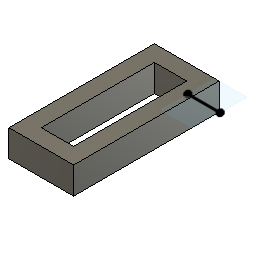
Teste+Medidor (Autodesk Fusion 360 design; units mm, degrees)
Autodesk Fusion 360 part; units mm, degrees
sketch "Esboço1" plane through (0, 0, 0) normal (0, 0, 1) x (1, 0, 0)
  line L0 (0, 0) -> (28.4, 0)
  line L1 (28.4, 0) -> (28.4, 58.2)
  line L2 (28.4, 58.2) -> (0, 58.2)
  line L3 (0, 58.2) -> (0, 0)
  line L4 (-5.0078, -5.0078) -> (33.4078, -5.0078)
  line L5 (33.4078, -5.0078) -> (33.4078, 63.2078)
  line L6 (33.4078, 63.2078) -> (-5.0078, 63.2078)
  line L7 (-5.0078, 63.2078) -> (-5.0078, -5.0078)
  dimension "d1" = 28.4
  dimension "d2" = 58.2
  dimension "d3" = 5.0078
  constraint horizontal L0
  constraint vertical L1
  constraint horizontal L2
  constraint vertical L3
  constraint coincident L0.start L3.end
  measures "d1" distance of L0.start L0.end
  measures "d2" distance of L0.start L2.end
extrude "Extrusão1" add sketch "Esboço1" along normal blind 10 makes body 1
sketch "Esboço2" plane through (0, 0, 0) normal (0, 1, 0) x (-1, 0, 0)
  line L0 (-28.4, 0) -> (0, 0)
  line L1 (0, 0) -> (0, 10)
  line L2 (0, 10) -> (-28.4, 10)
  line L3 (-28.4, 10) -> (-28.4, 0)
  line L4 (-14.2, 0) -> (-17.2, 0)
  line L5 (-17.2, 0) -> (-17.2, 10)
  line L6 (-17.2, 10) -> (-14.2, 10)
  line L7 (-14.2, 10) -> (-14.2, 0)
  line L8 (-14.2, 0) -> (-11.2, 0)
  line L9 (-11.2, 0) -> (-11.2, 10)
  line L10 (-11.2, 10) -> (-14.2, 10)
  line L11 (-14.2, 10) -> (-14.2, 0)
  dimension "d6" = 3
  constraint horizontal L4
  constraint vertical L5
  constraint horizontal L6
  constraint vertical L7
  constraint coincident L2 L5.end
  constraint midpoint L0 L4.start
  constraint horizontal L8
  constraint vertical L9
  constraint horizontal L10
  constraint vertical L11
  constraint coincident L2 L9.end
  measures "d6" distance of L4.start L4.end
extrude "Extrusão2" cut sketch "Esboço2" along normal blind -0.6 and the other way blind -58.8 contours L0 L2 L4 L5 L6 L7 L11 | L0 L2 L7 L8 L9 L10 L11 bodies 1
sketch "Esboço3" plane through (0, 58.8, 0) normal (0, -1, 0) x (1, 0, 0)
  line L0 (11.2, 0) -> (17.2, 0)
  line L1 (17.2, 0) -> (17.2, 10)
  line L2 (17.2, 10) -> (11.2, 10)
  line L3 (11.2, 10) -> (11.2, 0)
  line L4 (11.2, 5) -> (17.2, 5)
  line L5 (17.2, 4.9) -> (11.2, 4.9)
  line L6 (17.2, 5.1) -> (11.2, 5.1)
  line L7 (17.2, 5.1) -> (17.2, 4.9)
  line L8 (11.2, 5.1) -> (11.2, 4.9)
  dimension "d11" = 0.1
  dimension "d12" = 0.1
  constraint midpoint L3 L4.start
  constraint midpoint L1 L4.end
  constraint coincident L1 L5.start
  constraint coincident L3 L5.end
  constraint perpendicular L3 L5
  constraint coincident L1 L6.start
  constraint coincident L3 L6.end
  constraint perpendicular L3 L6
  measures "d11" distance of L4 L6
  measures "d12" distance of L4 L5
extrude "Extrusão4" cut sketch "Esboço3" against normal blind 0.3 contours L1 L3 L4 L5 L7 L8 | L1 L3 L4 L6 L7 L8 bodies 1
chamfer "Chanfro1" distance 1.2 distance2 0.3 2 edges at (14.2, 58.8, 5.1) (14.2, 58.8, 4.9) measured on face at (15.2, 58.8, 8.3667) measured on face at (15.2, 58.8, 3.2667) on bodies 1
sketch "Sketch5" plane through (0, 58.8, 0) normal (0, -1, 0) x (1, 0, 0)
  line L0 (0, 0) -> (12, 0)
  line L1 (12, 0) -> (12, 27)
  line L2 (12, 27) -> (0, 27)
  line L3 (0, 27) -> (0, 0)
  line L4 (9, 3) -> (3, 3)
  line L5 (3, 3) -> (3, 24)
  line L6 (3, 24) -> (9, 24)
  line L7 (9, 24) -> (9, 3)
  line L8 (9, 3) -> (3, 24) construction
  line L9 (3, 3) -> (9, 24) construction
  point P0 (6, 13.5)
  dimension "d25" = 12
  dimension "d26" = 27
  dimension "d27" = 6
  dimension "d28" = 21
  constraint horizontal L0
  constraint vertical L1
  constraint horizontal L2
  constraint vertical L3
  constraint coincident L0.start L3.end
  constraint horizontal L4
  constraint perpendicular L4 L5
  constraint parallel L4 L6
  constraint parallel L5 L7
  constraint coincident L8 P0
  constraint coincident L9 P0
  measures "d25" distance of L0.start L0.end
  measures "d26" distance of L0.start L2.end
  measures "d27" distance of L5.end L6.end
  measures "d28" distance of L4.end L5.end
extrude "Extrude6" add sketch "Sketch5" along normal blind 5 separate body makes body 2
sketch "Esboço4" plane through (0, -0.6, 0) normal (0, 1, 0) x (-1, 0, 0)
  line L0 (-17.2, 0) -> (-11.2, 0)
  line L1 (-11.2, 0) -> (-11.2, 10)
  line L2 (-11.2, 10) -> (-17.2, 10)
  line L3 (-17.2, 10) -> (-17.2, 0)
  line L4 (-11.2, 4.9) -> (-17.2, 4.9)
  line L5 (-11.2, 5.1) -> (-11.2, 4.9)
  line L6 (-11.2, 5.1) -> (-17.2, 5.1)
  line L7 (-17.2, 5) -> (-11.2, 5)
  line L8 (-17.2, 5.1) -> (-17.2, 4.9)
  dimension "d19" = 0.1
  dimension "d20" = 0.1
  measures "d19" distance of L6 L7
  measures "d20" distance of L4 L7
extrude "Extrusão5" [rolled back] along distance -0.3 taper angle 0
chamfer "Chanfro2" [rolled back] distance 1 1.2 distance 2 0.3
hidden bodies 1
